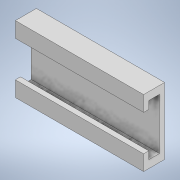
# Autodesk Inventor part: Part1_with_things
Saved by Autodesk Inventor 2021 (Build 250183000, 183)
## iProperties
Created: 2021-06-13
Part Number: Part1_with_things
Material: Generic
Document SubType Name: Modeling
Designer: user
Density: 1 g/cm^3
Appearance: Default
Author: user
Autodesk Inventor part; units mm, degrees
ref_plane "YZ Plane" through (0, 0, 0) normal (1, 0, 0) x (0, 1, 0)
ref_plane "XZ Plane" through (0, 0, 0) normal (0, 1, 0) x (-1, 0, 0)
ref_plane "XY Plane" through (0, 0, 0) normal (0, 0, 1) x (1, 0, 0)
sketch "Sketch1" plane through (0, 0, 0) normal (0, 0, 1) x (1, 0, 0)
  line L0 (-114.7642, 55) -> (135.2358, 55)
  line L1 (135.2358, 55) -> (135.2358, -75)
  line L2 (135.2358, -75) -> (-114.7642, -75)
  line L3 (-114.7642, -75) -> (-114.7642, 55)
  point P0 (0, 0)
  dimension "d0" = 250
  dimension "d1" = 130
  constraints: 8 end point, 2 parallel, 1 horizontal, 1 perpendicular
  measures "d0" distance of L0.start L0.end
  measures "d1" distance of L0.end L1.end
extrude "Extrusion1" add sketch "Sketch1" along normal blind 10
sketch "Sketch2" plane through (0, 0, 10) normal (0, 0, 1) x (1, 0, 0)
  line L0 (135.2358, 55) -> (-114.7642, 55) projected
  line L1 (135.2358, -75) -> (135.2358, 55) projected
  line L2 (-114.7642, 55) -> (135.2358, 55)
  line L3 (135.2358, 55) -> (135.2358, 40)
  line L4 (135.2358, 40) -> (-114.7642, 40)
  line L5 (-114.7642, 40) -> (-114.7642, 55)
  line L6 (-114.7642, -75) -> (135.2358, -75)
  line L7 (135.2358, -75) -> (135.2358, -60)
  line L8 (135.2358, -60) -> (-114.7642, -60)
  line L9 (-114.7642, -60) -> (-114.7642, -75)
  point P0 (0, 0)
  dimension "d4" = 15
  dimension "d5" = 15
  constraints: 16 end point, 4 parallel, 2 horizontal, 2 perpendicular, 2 point on line
  measures "d4" distance of L4.end L0.end
  measures "d5" distance of L8.end L6.start
extrude "Extrusion2" add sketch "Sketch2" along normal blind 21
sketch "Sketch3" plane through (0, 0, 31) normal (0, 0, 1) x (1, 0, 0)
  line L0 (-114.7642, 55) -> (-114.7642, -75) projected
  line L1 (135.2358, -60) -> (135.2358, 40) projected
  line L2 (-114.7642, 55) -> (135.2358, 55)
  line L3 (135.2358, 55) -> (135.2358, 25)
  line L4 (135.2358, 25) -> (-114.7642, 25)
  line L5 (-114.7642, 25) -> (-114.7642, 55)
  line L6 (135.2358, -75) -> (135.2358, -60) projected
  line L7 (135.2358, -75) -> (-114.7642, -75)
  line L8 (-114.7642, -75) -> (-114.7642, -45)
  line L9 (-114.7642, -45) -> (135.2358, -45)
  line L10 (135.2358, -45) -> (135.2358, -75)
  point P0 (0, 0)
  point P1 (-114.7642, -45)
  dimension "d8" = 30
  dimension "d9" = 30
  constraints: 16 end point, 4 parallel, 2 horizontal, 2 perpendicular, 2 point on line
  measures "d8" distance between parallel lines of L4 L2
  measures "d9" distance between parallel lines of L7 L9
extrude "Extrusion3" add sketch "Sketch3" along normal blind 10 contours L2 L3 L1 L4 L0 | L9 L1 L6 L7 L0
sketch "Sketch4" plane through (-114.7642, -75, 0) normal (-1, 0, 0) x (0, 0, 1)
  line L0 (7.1242, 110) -> (2.1242, 110)
  line L1 (2.1242, 110) -> (2.1242, 100)
  line L2 (2.1242, 100) -> (7.1242, 100)
  line L3 (7.1242, 100) -> (7.1242, 110)
  line L4 (7.1242, 30) -> (2.1242, 30)
  line L5 (2.1242, 30) -> (2.1242, 20)
  line L6 (2.1242, 20) -> (7.1242, 20)
  line L7 (7.1242, 20) -> (7.1242, 30)
  line L8 (31, 100) -> (41, 100) projected
  line L9 (31, 30) -> (41, 30) projected
  point P0 (0, 75)
  dimension "d12" = 5
  dimension "d13" = 10
  dimension "d14" = 10
  dimension "d15" = 0
  dimension "d16" = 0
  constraints: 16 end point, 4 parallel, 2 horizontal, 2 perpendicular, 2 point on line
  measures "d12" distance of L0.start L0.end
  measures "d13" distance of L2.end L0.start
  measures "d14" distance of L6.end L4.start
  measures "d15" distance between parallel lines of L8 L2
  measures "d16" distance between parallel lines of L9 L4
extrude "Extrusion4" cut sketch "Sketch4" against normal blind 20
equation "\"d5\" = d4"
equation "\"d9\" = d8"
body "Solid1"
